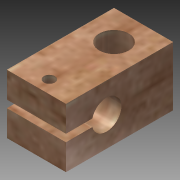
# Autodesk Inventor part: BarClamp_V3
Saved by Autodesk Inventor 2014 (Build 180170000, 170)
## iProperties
Created: 2013-12-27
Part Number: BarClamp_V3
Material: Birch
Document SubType Name: Modeling
Designer: Bram
Density: 0.512 g/cm^3
Appearance: Birch - Natural Medium Gloss
Author: Bram
Autodesk Inventor part; units mm, degrees
ref_plane "YZ Plane" through (0, 0, 0) normal (1, 0, 0) x (0, 1, 0)
ref_plane "XZ Plane" through (0, 0, 0) normal (0, 1, 0) x (-1, 0, 0)
ref_plane "XY Plane" through (0, 0, 0) normal (0, 0, 1) x (1, 0, 0)
sketch "Sketch1" plane through (0, 0, 0) normal (0, 1, 0) x (-1, 0, 0)
  line L0 (0, 0) -> (16, 0)
  line L1 (16, 0) -> (16, 16)
  line L2 (16, 16) -> (0, 16)
  line L3 (0, 16) -> (0, 0)
  dimension "d0" = 16
  dimension "d1" = 16
  constraints: 8 end point, 2 parallel, 1 horizontal, 1 perpendicular
  measures "d0" distance of L2.end L1.end
  measures "d1" distance of L1.end L0.end
extrude "Extrusion1" add sketch "Sketch1" along normal blind 29
sketch "Sketch2" plane through (-16, 0, 16) normal (0, 0, 1) x (1, 0, 0)
  circle A0 centre (8, 3.5) radius 1.5
  circle A1 centre (8, 21) radius 4
  dimension "d5" = 3
  dimension "d7" = 8
  constraints: 2 centre point
  measures "d5" diameter of A0
  measures "d7" diameter of A1
extrude "Extrusion2" cut sketch "Sketch2" against normal blind 29
sketch "Sketch3" plane through (0, 0, 16) normal (1, 0, 0) x (0, 0, -1)
  line L0 (0, 0) -> (16, 0) projected
  line L1 (16, 0) -> (16, 29) projected
  line L2 (0, 0) -> (0, 29) projected
  line L3 (0, 0) -> (0, 11)
  arc A0 (9, 7.127) -> (7, 7.127) centre (8, 11) ccw
  line L4 (8, 0) -> (9, 0)
  line L5 (9, 0) -> (9, 7.127)
  line L6 (8, 0) -> (7, 0)
  line L7 (7, 0) -> (7, 7.127)
  line L8 (0, 11) -> (4, 11)
  line L9 (12, 11) -> (16, 11)
  dimension "d10" = 11
  dimension "d11" = 8
  dimension "d12" = 1
  dimension "d13" = 1
  constraints: 14 end point, 4 perpendicular, 4 point on circle, 4 point on line, 1 centre point, 1 midpoint
  measures "d10" distance of L0.start L3.end
  measures "d11" diameter of A0
  measures "d12" distance of L4.start L4.end
  measures "d13" distance of L4.start L6.end
extrude "Extrusion3" cut sketch "Sketch3" against normal blind 29 contours L7 A0 L5 L0
body "Solid1"
